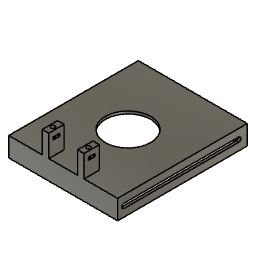
base brazo elevador (Autodesk Fusion 360 design; units mm, degrees)
Autodesk Fusion 360 part; units mm, degrees
sketch "Sketch1" plane through (0, 0, 0) normal (0, 0, 1) x (1, 0, 0)
  line L0 (0, 0) -> (84, 0)
  line L1 (84, 0) -> (84, 100)
  line L2 (84, 100) -> (0, 100)
  line L3 (0, 100) -> (0, 0)
  dimension "d1" = 84
  dimension "d2" = 100
  constraint horizontal L0
  constraint vertical L1
  constraint horizontal L2
  constraint vertical L3
  constraint coincident L0.start L3.end
  measures "d1" distance of L0.start L0.end
  measures "d2" distance of L0.start L2.end
extrude "Extrude1" add sketch "Sketch1" along normal blind 15
shell "Shell1" thickness 2 removed faces 1 at (28, 66.6667, 0)
sketch "Sketch2" plane through (84, 0, 0) normal (1, 0, 0) x (0, 1, 0)
  line L0 (0, 0) -> (100, 0)
  line L1 (100, 0) -> (100, 15)
  line L2 (100, 15) -> (0, 15)
  line L3 (0, 15) -> (0, 0)
  line L4 (0, 7.5) -> (5, 7.5)
  line L5 (100, 7.5) -> (98.4347, 7.5)
  line L6 (98.4347, 7.5) -> (93.4347, 7.5)
  circle A0 centre (5, 7.5) radius 1.75
  circle A1 centre (93.4347, 7.5) radius 1.75
  line L7 (5, 9.25) -> (93.4347, 9.25)
  line L8 (5, 5.75) -> (93.4347, 5.75)
  dimension "d6" = 5
  dimension "d7" = 5
  dimension "d8" = 3.5
  dimension "d9" = 3.5
  constraint midpoint L3 L4.start
  constraint perpendicular L3 L4
  constraint midpoint L1 L5.start
  constraint perpendicular L1 L5
  constraint perpendicular L1 L6
  constraint coincident L4.end A0.centre
  constraint coincident L6.end A1.centre
  constraint coincident A0 L7.start
  constraint coincident A1 L7.end
  constraint tangent A1 L7
  constraint parallel L4 L7
  constraint coincident A0 L8.start
  constraint coincident A1 L8.end
  constraint tangent A1 L8
  constraint parallel L7 L8
  measures "d6" distance of L4.start L4.end
  measures "d7" distance of L5.end L6.end
  measures "d8" diameter of A0
  measures "d9" diameter of A1
extrude "Extrude2" cut sketch "Sketch2" against normal blind 225 contours A0 | A0 A1 L7 L8 | A1
sketch "Sketch3" plane through (0, 0, 15) normal (0, 0, 1) x (-1, 0, 0)
  line L0 (0, -100) -> (0, 0)
  line L1 (0, 0) -> (-84, 0)
  line L2 (-84, 0) -> (-84, -100)
  line L3 (-84, -100) -> (0, -100)
  circle A0 centre (-42, -50) radius 17.5
  dimension "d12" = 35
  measures "d12" diameter of A0
extrude "Extrude3" cut sketch "Sketch3" against normal blind 30 contours A0
sketch "Sketch4" plane through (0, 0, 15) normal (0, 0, 1) x (-1, 0, 0)
  circle A0 centre (-42, -50) radius 17.5
  line L0 (0, -100) -> (0, 0)
  line L1 (0, 0) -> (-84, 0)
  line L2 (-84, 0) -> (-84, -100)
  line L3 (-84, -100) -> (0, -100)
  line L4 (-42, 0) -> (-42, -10)
  line L5 (-42, 0) -> (-58.1, 0)
  line L6 (-58.1, 0) -> (-58.1, -11.8)
  line L7 (-58.1, -11.8) -> (-25.9, -11.8)
  line L8 (-25.9, -11.8) -> (-25.9, 0)
  line L9 (-25.9, 0) -> (-30.9, 0)
  line L10 (-30.9, 0) -> (-30.9, -11.8)
  line L11 (-58.1, 0) -> (-58.1, -11.8)
  line L12 (-58.1, -11.8) -> (-53.1, -11.8)
  line L13 (-53.1, -11.8) -> (-53.1, 0)
  dimension "d15" = 16.1
  dimension "d16" = 11.8
  dimension "d17" = 32.2
  dimension "d18" = 5
  dimension "d19" = 5
  constraint midpoint L1 L4.start
  constraint perpendicular L1 L4
  constraint perpendicular L4 L5
  constraint perpendicular L5 L6
  constraint perpendicular L6 L7
  constraint coincident L1 L8.end
  constraint perpendicular L1 L8
  constraint perpendicular L8 L9
  constraint coincident L7 L10.end
  constraint perpendicular L7 L10
  constraint perpendicular L6 L12
  constraint vertical L13
  constraint coincident L5 L13.end
  measures "d15" distance of L4.start L5.end
  measures "d16" distance of L5.end L6.end
  measures "d17" distance of L6.end L7.end
  measures "d18" distance of L8.end L9.end
  measures "d19" distance of L6.end L12.end
extrude "Extrude4" add sketch "Sketch4" along normal blind 17 contours L1 L7 L8 L9 L10 | L1 L5 L6 L7 L11 L12 L13
sketch "Sketch5" plane through (0, 0, 32) normal (0, 0, 1) x (-1, 0, 0)
  line L0 (-30.9, 0) -> (-30.9, -11.8)
  line L1 (-30.9, -11.8) -> (-25.9, -11.8)
  line L2 (-25.9, -11.8) -> (-25.9, 0)
  line L3 (-25.9, 0) -> (-30.9, 0)
  circle A0 centre (-28.4, -5.9) radius 1.5
  dimension "d22" = 3
  measures "d22" diameter of A0
sketch "Sketch6" plane through (0, 0, 32) normal (0, 0, 1) x (-1, 0, 0)
  line L0 (-53.1, -11.8) -> (-53.1, 0)
  line L1 (-53.1, 0) -> (-58.1, 0)
  line L2 (-58.1, 0) -> (-58.1, -11.8)
  line L3 (-58.1, -11.8) -> (-53.1, -11.8)
  circle A0 centre (-55.6, -5.9) radius 1.5
  dimension "d23" = 3
  measures "d23" diameter of A0
extrude "Extrude5" cut sketch "Sketch6" sketch "Sketch5" against normal blind 12 contours A0 of sketch 2 contours A0
sketch "Sketch7" plane through (30.9, 0, 0) normal (1, 0, 0) x (0, 1, 0)
  line L0 (0, 15) -> (11.8, 15)
  line L1 (11.8, 15) -> (11.8, 32)
  line L2 (11.8, 32) -> (0, 32)
  line L3 (0, 32) -> (0, 15)
  line L4 (8.4, 27.7438) -> (3.4, 27.7438)
  line L5 (3.4, 27.7438) -> (3.4, 25.7438)
  line L6 (3.4, 25.7438) -> (8.4, 25.7438)
  line L7 (8.4, 25.7438) -> (8.4, 27.7438)
  line L8 (8.4, 27.7438) -> (3.4, 25.7438) construction
  line L9 (3.4, 27.7438) -> (8.4, 25.7438) construction
  point P0 (5.9, 26.7438)
  dimension "d26" = 5
  dimension "d27" = 2
  constraint horizontal L4
  constraint perpendicular L4 L5
  constraint parallel L4 L6
  constraint parallel L5 L7
  constraint coincident L8 P0
  constraint coincident L9 P0
  measures "d26" distance of L5.end L6.end
  measures "d27" distance of L4.end L5.end
extrude "Extrude6" cut sketch "Sketch7" along normal blind -5 and the other way blind -34 contours L4 L5 L6 L7
